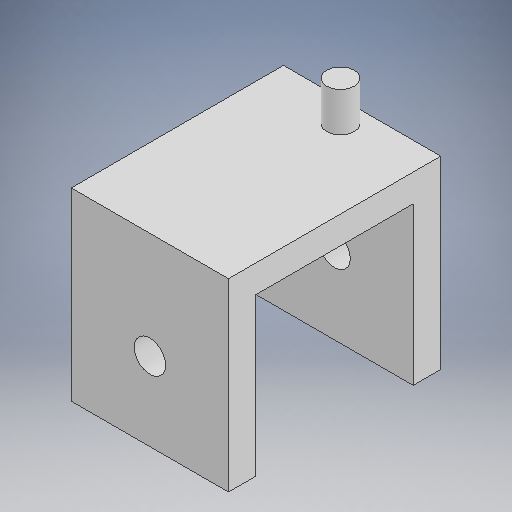
# Autodesk Inventor part: camera_case_jbh
Saved by Autodesk Inventor 2025.2 (Build 292293000, 293)
## iProperties
Created: 2025-03-10
Part Number: camera_case_jbh
Material: 일반
Document SubType Name: Modeling
Designer: jbhma
Density: 1 g/cm^3
Appearance: 기본값
Author: jbhma
Autodesk Inventor part; units mm, degrees
ref_plane "YZ Plane" through (0, 0, 0) normal (1, 0, 0) x (0, 1, 0)
ref_plane "XZ Plane" through (0, 0, 0) normal (0, 1, 0) x (-1, 0, 0)
ref_plane "XY Plane" through (0, 0, 0) normal (0, 0, 1) x (1, 0, 0)
sketch "스케치1" plane through (0, 0, 0) normal (0, 1, 0) x (-1, 0, 0)
  line L0 (0, 0) -> (-40, 0)
  line L1 (-40, 0) -> (-40, -54)
  line L2 (-40, -54) -> (0, -54)
  line L3 (0, -54) -> (0, 0)
  line L4 (0, 0) -> (-40, 0)
  line L5 (-40, 0) -> (-40, -7)
  line L6 (-40, -7) -> (0, -7)
  line L7 (0, -7) -> (0, 0)
  line L8 (-40, -54) -> (0, -54)
  line L9 (0, -54) -> (0, -47)
  line L10 (0, -47) -> (-40, -47)
  line L11 (-40, -47) -> (-40, -54)
  dimension "d0" = 40
  dimension "d1" = 54
  dimension "d2" = 40
  dimension "d3" = 7
  dimension "d4" = 40
  dimension "d5" = 7
  constraints: 24 end point, 6 parallel, 3 horizontal, 3 perpendicular
  measures "d0" distance of L2.end L1.end
  measures "d1" distance of L1.end L0.end
  measures "d2" distance of L6.end L5.end
  measures "d3" distance of L5.end L4.end
  measures "d4" distance of L10.end L9.end
  measures "d5" distance of L9.end L8.end
extrude "돌출1" add sketch "스케치1" along normal blind 7
sketch "스케치2" plane through (0, 0, 0) normal (0, -1, 0) x (1, 0, 0)
  line L0 (0, 0) -> (40, 0)
  line L1 (40, 0) -> (40, -7)
  line L2 (40, -7) -> (0, -7)
  line L3 (0, -7) -> (0, 0)
  line L4 (0, -54) -> (40, -54)
  line L5 (40, -54) -> (40, -47)
  line L6 (40, -47) -> (0, -47)
  line L7 (0, -47) -> (0, -54)
  dimension "d8" = 40
  dimension "d9" = 7
  dimension "d10" = 40
  dimension "d11" = 7
  constraints: 16 end point, 4 parallel, 2 horizontal, 2 perpendicular
  measures "d8" distance of L1.end L2.end
  measures "d9" distance of L0.end L1.end
  measures "d10" distance of L6.end L5.end
  measures "d11" distance of L5.end L4.end
extrude "돌출2" add sketch "스케치2" along normal blind 40
sketch "스케치9" plane through (0, 7, 0) normal (0, 0, 1) x (1, 0, 0)
  circle A0 centre (20, -27.074) radius 4
  point P0 (0, -7)
  dimension "d26" = 8
  constraints: 1 centre point
  measures "d26" diameter of A0
extrude "돌출6" cut sketch "스케치9" against normal blind 7
sketch "스케치10" plane through (0, 7, 0) normal (0, 1, 0) x (1, 0, 0)
  circle A0 centre (20.0781, 48.4236) radius 3.5197
  point P0 (0, 0)
  constraints: 1 centre point
extrude "돌출7" add sketch "스케치10" along normal blind 10
sketch "스케치11" plane through (40, 7, -54) normal (0, 0, -1) x (-1, 0, 0)
  circle A0 centre (20, -27.074) radius 4
  line L0 (40, -47) -> (0, -47) projected
  line L1 (0, -47) -> (0, 0) projected
  point P0 (40, -7)
  point P1 (20, -47)
  dimension "d31" = 8
  dimension "d32" = 19.926
  dimension "d33" = 20
  constraints: 1 centre point, 1 midpoint
  measures "d31" diameter of A0
  measures "d32" distance of A0.centre point (20, -47)
  measures "d33" distance from line of A0.centre L1
extrude "돌출8" cut sketch "스케치11" against normal blind 10
